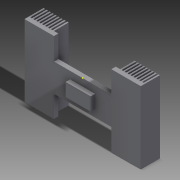
# Autodesk Inventor part: SensorCooler01
Saved by Autodesk Inventor 2015 (Build 190159000, 159)
## iProperties
Created: 2015-03-10
Part Number: SensorCooler01
Material: Generic
Document SubType Name: Modeling
Designer: spichelh
Density: 1 g/cm^3
Appearance: Default
Author: spichelh
Autodesk Inventor part; units mm, degrees
ref_plane "YZ Plane" through (0, 0, 0) normal (1, 0, 0) x (0, 1, 0)
ref_plane "XZ Plane" through (0, 0, 0) normal (0, 1, 0) x (-1, 0, 0)
ref_plane "XY Plane" through (0, 0, 0) normal (0, 0, 1) x (1, 0, 0)
sketch "Sketch2" plane through (0, 0, 0) normal (0, 0, 1) x (1, 0, 0)
  line L0 (-8.5, 4.5) -> (8.5, 4.5)
  line L1 (8.5, 4.5) -> (8.5, -4.5)
  line L2 (8.5, -4.5) -> (-8.5, -4.5)
  line L3 (-8.5, -4.5) -> (-8.5, 4.5)
  line L4 (8.5, 4.5) -> (-8.5, -4.5) construction
  line L5 (8.5, -4.5) -> (-8.5, 4.5) construction
  point P0 (0, 0)
  dimension "d12" = 17
  dimension "d13" = 9
  constraints: 12 end point, 2 midpoint, 2 parallel, 1 horizontal, 1 perpendicular
  measures "d12" distance of L1.end L2.end
  measures "d13" distance of L0.end L1.end
extrude "Extrusion2" add sketch "Sketch2" along normal blind 3
sketch "Sketch3" plane through (0, 0, 0) normal (0, 0, -1) x (-1, 0, 0)
  line L0 (-19.5, 9.5) -> (19.5, 9.5)
  line L1 (19.5, 9.5) -> (19.5, -9.5)
  line L2 (19.5, -9.5) -> (-19.5, -9.5)
  line L3 (-19.5, -9.5) -> (-19.5, 9.5)
  line L4 (-19.5, 9.5) -> (19.5, -9.5) construction
  line L5 (19.5, 9.5) -> (-19.5, -9.5) construction
  line L6 (8.5, 4.5) -> (-8.5, 4.5) projected
  line L7 (-8.5, 4.5) -> (-8.5, -4.5) projected
  line L8 (19.5, 15) -> (-19.5, 15) construction
  line L9 (-19.5, 15) -> (-19.5, -15) construction
  line L10 (-19.5, -15) -> (19.5, -15) construction
  line L11 (19.5, -15) -> (19.5, 15) construction
  line L12 (19.5, -15) -> (-19.5, 15) construction
  line L13 (-19.5, -15) -> (19.5, 15) construction
  line L14 (-19.5, 24.5) -> (-39.5, 24.5)
  line L15 (-19.5, 9.5) -> (-19.5, 24.5)
  line L16 (-39.5, 24.5) -> (-39.5, 0)
  line L17 (0, 0) -> (15.34, 0) construction
  line L18 (-19.5, -24.5) -> (-39.5, -24.5)
  line L19 (-19.5, -9.5) -> (-19.5, -24.5)
  line L20 (-39.5, -24.5) -> (-39.5, 0)
  line L21 (0, 0) -> (0, 17) construction
  line L22 (19.5, 24.5) -> (39.5, 24.5)
  line L23 (19.5, 9.5) -> (19.5, 24.5)
  line L24 (39.5, 24.5) -> (39.5, 0)
  line L25 (19.5, -9.5) -> (19.5, -24.5)
  line L26 (19.5, -24.5) -> (39.5, -24.5)
  line L27 (39.5, -24.5) -> (39.5, 0)
  dimension "d16" = 11
  dimension "d17" = 5
  dimension "d18" = 39
  dimension "d39" = 19
  dimension "d55" = 39
  dimension "d56" = 30
  dimension "d57" = 15
  dimension "d58" = 20
  dimension "d78" = 49
  constraints: 52 end point, 7 symmetric about line, 6 midpoint, 5 parallel, 3 horizontal, 3 perpendicular, 2 vertical
  measures "d16" distance between parallel lines of L3 L7
  measures "d17" distance between parallel lines of L0 L6
  measures "d18" distance between parallel lines of L1 L3
  measures "d39" distance between parallel lines of L2 L0
  measures "d55" distance of L10.end L9.end
  measures "d56" distance of L9.end L8.end
  measures "d57" distance between parallel lines of L14 L0
  measures "d58" distance between parallel lines of L15 L16
  measures "d78" distance between parallel lines of L14 L18
extrude "Extrusion3" add sketch "Sketch3" along normal blind 3
sketch "Sketch6" plane through (-19.5, 9.5, 0) normal (0, 1, 0) x (1, 0, 0)
  point P0 (19.5, 0)
sketch "Sketch7" plane through (19.5, 24.5, 0) normal (0, 1, 0) x (1, 0, 0)
  line L0 (20, 3) -> (20, 13)
  line L1 (20, 13) -> (19, 13)
  line L2 (19, 13) -> (19, 3)
  line L3 (-19.5, 0) -> (-19.5, 8) construction
  line L4 (20, 3) -> (19, 3)
  line L5 (18, 3) -> (18, 13)
  line L6 (18, 13) -> (17, 13)
  line L7 (17, 13) -> (17, 3)
  line L8 (18, 3) -> (17, 3)
  line L9 (16, 3) -> (16, 13)
  line L10 (16, 13) -> (15, 13)
  line L11 (15, 13) -> (15, 3)
  line L12 (16, 3) -> (15, 3)
  line L13 (14, 3) -> (14, 13)
  line L14 (14, 13) -> (13, 13)
  line L15 (13, 13) -> (13, 3)
  line L16 (14, 3) -> (13, 3)
  line L17 (12, 3) -> (12, 13)
  line L18 (12, 13) -> (11, 13)
  line L19 (11, 13) -> (11, 3)
  line L20 (12, 3) -> (11, 3)
  line L21 (10, 3) -> (10, 13)
  line L22 (10, 13) -> (9, 13)
  line L23 (9, 13) -> (9, 3)
  line L24 (10, 3) -> (9, 3)
  line L25 (8, 3) -> (8, 13)
  line L26 (8, 13) -> (7, 13)
  line L27 (7, 13) -> (7, 3)
  line L28 (8, 3) -> (7, 3)
  line L29 (6, 3) -> (6, 13)
  line L30 (6, 13) -> (5, 13)
  line L31 (5, 13) -> (5, 3)
  line L32 (6, 3) -> (5, 3)
  line L33 (4, 3) -> (4, 13)
  line L34 (4, 13) -> (3, 13)
  line L35 (3, 13) -> (3, 3)
  line L36 (4, 3) -> (3, 3)
  line L37 (0, 0) -> (-39, 0) projected
  line L38 (-59, 3) -> (-59, 13)
  line L39 (-59, 13) -> (-58, 13)
  line L40 (-58, 13) -> (-58, 3)
  line L41 (-59, 3) -> (-58, 3)
  line L42 (-57, 3) -> (-57, 13)
  line L43 (-57, 13) -> (-56, 13)
  line L44 (-56, 13) -> (-56, 3)
  line L45 (-57, 3) -> (-56, 3)
  line L46 (-55, 3) -> (-55, 13)
  line L47 (-55, 13) -> (-54, 13)
  line L48 (-54, 13) -> (-54, 3)
  line L49 (-55, 3) -> (-54, 3)
  line L50 (-53, 3) -> (-53, 13)
  line L51 (-53, 13) -> (-52, 13)
  line L52 (-52, 13) -> (-52, 3)
  line L53 (-53, 3) -> (-52, 3)
  line L54 (-51, 3) -> (-51, 13)
  line L55 (-51, 13) -> (-50, 13)
  line L56 (-50, 13) -> (-50, 3)
  line L57 (-51, 3) -> (-50, 3)
  line L58 (-49, 3) -> (-49, 13)
  line L59 (-49, 13) -> (-48, 13)
  line L60 (-48, 13) -> (-48, 3)
  line L61 (-49, 3) -> (-48, 3)
  line L62 (-47, 3) -> (-47, 13)
  line L63 (-47, 13) -> (-46, 13)
  line L64 (-46, 13) -> (-46, 3)
  line L65 (-47, 3) -> (-46, 3)
  line L66 (-45, 3) -> (-45, 13)
  line L67 (-45, 13) -> (-44, 13)
  line L68 (-44, 13) -> (-44, 3)
  line L69 (-45, 3) -> (-44, 3)
  line L70 (-43, 3) -> (-43, 13)
  line L71 (-43, 13) -> (-42, 13)
  line L72 (-42, 13) -> (-42, 3)
  line L73 (-43, 3) -> (-42, 3)
  dimension "d59" = 10
  dimension "d60" = 1
  dimension "d71" = 2
  dimension "d76" = 79
  dimension "d77" = 3
  constraints: 146 end point, 36 symmetric about line, 2 perpendicular, 2 vertical, 1 collinear, 1 horizontal, 63 other
  measures "d59" distance of L0.start L0.end
  measures "d60" distance of L0.end L1.end
  measures "d71" distance of L0.end L5.end
  measures "d76" diameter of L0.start L3
  measures "d77" distance from line of L0.start L37
extrude "Extrusion6" add sketch "Sketch7" against normal blind 49
body "Solid2"
